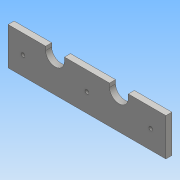
# Autodesk Inventor part: Pinhole_insert_1mm_3x
Saved by Autodesk Inventor 2016 (Build 200138000, 138)
## iProperties
Created: 2016-03-11
Part Number: Pinhole_insert_1mm_3x
Material: Generic
Document SubType Name: Modeling
Designer: admin
Density: 1 g/cm^3
Appearance: Default
Author: admin
Autodesk Inventor part; units mm, degrees
ref_plane "YZ Plane" through (0, 0, 0) normal (1, 0, 0) x (0, 1, 0)
ref_plane "XZ Plane" through (0, 0, 0) normal (0, 1, 0) x (-1, 0, 0)
ref_plane "XY Plane" through (0, 0, 0) normal (0, 0, 1) x (1, 0, 0)
sketch "Sketch1" plane through (0, 0, 0) normal (0, 1, 0) x (-1, 0, 0)
  line L0 (21, 5) -> (-21, 5)
  line L1 (-21, 5) -> (-21, -5)
  line L2 (-21, -5) -> (21, -5)
  line L3 (21, -5) -> (21, 5)
  point P0 (0, 0)
  point P1 (21, 0)
  point P2 (0, -5)
  point P3 (17, 0)
  point P4 (0, 0)
  point P5 (-17, 0)
  dimension "d0" = 42
  dimension "d1" = 10
  dimension "d2" = 17
  dimension "d3" = 17
  constraints: 8 end point, 4 horizontal alignment, 2 midpoint, 2 parallel, 1 coincident, 1 horizontal, 1 perpendicular, 1 vertical alignment
  measures "d0" distance of L0.start L0.end
  measures "d1" distance of L2.end L0.start
  measures "d2" distance of point (0, 0) point (17, 0)
  measures "d3" distance of point (-17, 0) point (0, 0)
extrude "Extrusion1" add sketch "Sketch1" along normal blind 1.6
sketch "Sketch2" plane through (0, 1.6, 0) normal (0, 1, 0) x (1, 0, 0)
  point P0 (0, 0)
  point P1 (-17, 0)
  point P2 (0, 0)
  point P3 (17, 0)
hole "Hole1" at (-17, 1.6, 0) at (0, 1.6, 0) at (17, 1.6, 0) direction (0, -1, 0) diameter 1 end through all
sketch "Sketch3" plane through (0, 1.6, 0) normal (0, 1, 0) x (1, 0, 0)
  line L0 (-21, -5) -> (21, -5) projected
  line L1 (-21, -5) -> (21, -5) projected
  line L2 (-8.5, 0.5052) -> (-8.5, -1.9497) construction
  line L3 (8.5, -1.3927) -> (8.5, 1.0622) construction
  arc A0 (-6, -4) -> (-11, -4) centre (-8.5, -4) ccw
  arc A1 (11, -4) -> (6, -4) centre (8.5, -4) ccw
  line L4 (-11, -4) -> (-11, -5)
  line L5 (-6, -4) -> (-6, -5)
  line L6 (6, -4) -> (6, -5)
  line L7 (11, -4) -> (11, -5)
  point P0 (0, 0)
  dimension "d15" = 17
  dimension "d16" = 8.5
  dimension "d21" = 5
  dimension "d22" = 1
  constraints: 12 end point, 6 point on line, 4 perpendicular, 4 point on circle, 4 tangent, 2 centre point, 2 vertical, 1 equal radius, 1 horizontal alignment
  measures "d15" distance between parallel lines of L3 L2
  measures "d16" distance from line of L2 point (0, 0)
  measures "d21" diameter of A0
  measures "d22" distance from line of L0 A0.centre
extrude "Extrusion2" cut sketch "Sketch3" against normal blind 1.6
equation "\"d3\" = d2"
body "Solid1"
